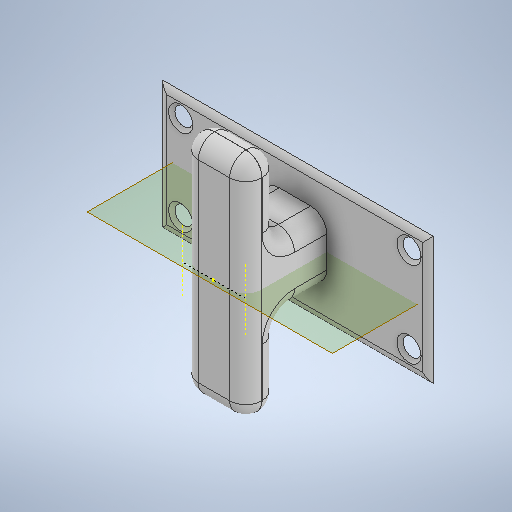
# Autodesk Inventor part: WireWrappoMatica(TM)
Saved by Autodesk Inventor 2025.1 (Build 291241000, 241)
## iProperties
Created: 2024-10-25
Part Number: WireWrappoMatica(TM)
Material: Generic
Document SubType Name: Modeling
Designer: ishaa
Density: 1 g/cm^3
Appearance: Default
Author: ishaa
Autodesk Inventor part; units mm, degrees
ref_plane "YZ Plane" through (0, 0, 0) normal (1, 0, 0) x (0, 1, 0)
ref_plane "XZ Plane" through (0, 0, 0) normal (0, 1, 0) x (-1, 0, 0)
ref_plane "XY Plane" through (0, 0, 0) normal (0, 0, 1) x (1, 0, 0)
sketch "Sketch1" plane through (0, 0, 0) normal (0, 0, 1) x (1, 0, 0)
  line L0 (-42.5, -20) -> (42.5, -20)
  line L1 (42.5, -20) -> (42.5, 20)
  line L2 (42.5, 20) -> (-42.5, 20)
  line L3 (-42.5, 20) -> (-42.5, -20)
  line L4 (-42.5, -20) -> (42.5, 20) construction
  line L5 (42.5, -20) -> (-42.5, 20) construction
  point P0 (0, 0)
  dimension "d0" = 85
  dimension "d1" = 40
  constraints: 12 end point, 2 midpoint, 2 parallel, 1 horizontal, 1 perpendicular
  measures "d0" distance of L2.end L1.end
  measures "d1" distance of L1.end L0.end
extrude "Extrusion1" add sketch "Sketch1" along normal blind 1
fillet "Fillet1" radius 3.175 4 edges at (-42.5, 0, 1) (0, 20, 1) (0, -20, 1) (42.5, 0, 1)
sketch "Sketch2" plane through (0, 0, 1) normal (0, 0, 1) x (1, 0, 0)
  line L0 (-40.187, -17.687) -> (-40.187, 17.687) construction
  line L1 (-40.187, 0) -> (40.187, 0) construction
  line L2 (40.187, 17.687) -> (40.187, -17.687) construction
  line L3 (-40.187, 17.687) -> (40.187, 17.687) construction
  line L4 (0, 17.687) -> (0, -17.687) construction
  line L5 (40.187, -17.687) -> (-40.187, -17.687) construction
  line L6 (10, -10) -> (-10, -10)
  line L7 (-10, -10) -> (-10, 10)
  line L8 (-10, 10) -> (10, 10)
  line L9 (10, 10) -> (10, -10)
  line L10 (10, -10) -> (-10, 10) construction
  line L11 (-10, -10) -> (10, 10) construction
  point P0 (0, 0)
  dimension "d5" = 20
  dimension "d6" = 20
  constraints: 16 end point, 6 midpoint, 2 parallel, 1 horizontal, 1 perpendicular
  measures "d5" distance of L7.end L8.end
  measures "d6" distance of L6.end L7.end
extrude "Extrusion2" add sketch "Sketch2" along normal blind 25.4
sketch "Sketch3" plane through (-10, -10, 1) normal (0, -1, 0) x (1, 0, 0)
  line L0 (20, 25.4) -> (0, 25.4) projected
  line L1 (20, 0) -> (20, 25.4) projected
  line L2 (0, 25.4) -> (20, 25.4)
  line L3 (20, 25.4) -> (20, 15.1947)
  line L4 (20, 15.1947) -> (0, 15.1947)
  line L5 (0, 15.1947) -> (0, 25.4)
  point P0 (10, -1)
  constraints: 8 end point, 2 parallel, 1 horizontal, 1 perpendicular, 1 point on line
sketch "Sketch4" plane through (0, 0, 26.4) normal (0, 0, 1) x (1, 0, 0)
  line L0 (-10, -10) -> (-10, 10) construction
  line L1 (-10, 0) -> (10, 0) construction
  line L2 (10, 10) -> (10, -10) construction
  point P0 (0, 0)
  constraints: 2 end point, 2 midpoint
ref_plane "Work Plane1" through (-10, 0, 26.4) normal (0, -1, 0) x (1, 0, 0)
extrude "Extrusion3" add sketch "Sketch3" along normal blind 25.4
mirror "Mirror1" about plane through (-10, 0, 26.4) normal (0, -1, 0) of "Extrusion3"
fillet "Fillet2" radius 5.08 2 edges at (0, -10, 16.1947) (0, 10, 16.1947)
fillet "Fillet3" radius 5.08 22 edges at (-10, 35.4, 21.2974) (10, 35.4, 21.2974) (0, 35.4, 16.1947) (0, 35.4, 26.4) (-10, 0, 26.4) (-10, -35.4, 21.2974) (10, -35.4, 21.2974) (10, 0, 26.4) (10, 11.4879, 14.7068) (10, 10, 6.0574) (10, 25.24, 16.1947) (-10, 11.4879, 14.7068) (-10, 10, 6.0574) (-10, 25.24, 16.1947) (-10, -11.4879, 14.7068) (-10, -10, 6.0574) (-10, -25.24, 16.1947) (0, -35.4, 16.1947) (10, -11.4879, 14.7068) (10, -10, 6.0574) (10, -25.24, 16.1947) (0, -35.4, 26.4)
sketch "Sketch5" plane through (0, 0, 1) normal (0, 0, 1) x (1, 0, 0)
  circle A0 centre (-35.8589, 13.4243) radius 2.8
  line L0 (59.5, 0) -> (-59.5, 0) projected
  line L1 (10, 4.92) -> (10, -4.92) projected
  arc A1 (4.92, -10) -> (10, -4.92) centre (4.92, -4.92) ccw projected
  line L2 (4.92, -10) -> (-4.92, -10) projected
  arc A2 (-10, -4.92) -> (-4.92, -10) centre (-4.92, -4.92) ccw projected
  line L3 (-10, -4.92) -> (-10, 4.92) projected
  arc A3 (-4.92, 10) -> (-10, 4.92) centre (-4.92, 4.92) ccw projected
  line L4 (-4.92, 10) -> (4.92, 10) projected
  arc A4 (10, 4.92) -> (4.92, 10) centre (4.92, 4.92) ccw projected
  line L5 (40.187, 17.687) -> (40.187, -17.687) projected
  line L6 (-40.187, 17.687) -> (40.187, 17.687) projected
  line L7 (-40.187, -17.687) -> (-40.187, 17.687) projected
  line L8 (40.187, -17.687) -> (-40.187, -17.687) projected
  circle A5 centre (-35.8589, -13.4243) radius 2.8
  line L9 (42.5, 20) -> (-42.5, 20) construction
  line L10 (0, 20) -> (0, -20) construction
  line L11 (-42.5, -20) -> (42.5, -20) construction
  circle A6 centre (35.8589, 13.4243) radius 2.8
  circle A7 centre (35.8589, -13.4243) radius 2.8
  point P0 (0, 0)
  dimension "d14" = 5.6
  constraints: 4 centre point, 3 symmetric about line, 2 end point, 2 midpoint, 3 other
  measures "d14" diameter of A0
extrude "Extrusion4" cut sketch "Sketch5" against normal blind 345.1324 contours A0 | A5 | A6 | A7
chamfer "Chamfer1" distance 1 angle 45 4 edges at (33.0589, 13.4243, 1) (33.0589, -13.4243, 1) (-38.6589, 13.4243, 1) (-38.6589, -13.4243, 1)
body "Solid1"
